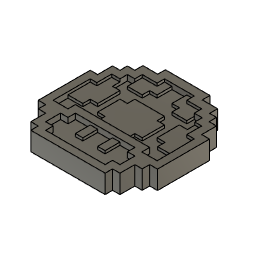
mushroom-8-bit (Autodesk Fusion 360 design; units mm, degrees)
Autodesk Fusion 360 part; units mm, degrees
sketch "Limit" plane through (0, 0, 0) normal (0, 0, 1) x (1, 0, 0)
  line L0 (0, 0) -> (70, 0)
  line L1 (70, 0) -> (70, 100)
  line L2 (70, 100) -> (0, 100)
  line L3 (0, 100) -> (0, 0)
  constraint horizontal L0
  constraint vertical L1
  constraint horizontal L2
  constraint vertical L3
  constraint coincident L0.start L3.end
sketch "Mushroom Head" plane through (0, 0, 0) normal (0, 0, 1) x (1, 0, 0)
  line L0 (11, 35) -> (11, 27)
  line L1 (11, 27) -> (15, 27)
  line L2 (15, 27) -> (15, 23)
  line L3 (15, 23) -> (55, 23)
  line L4 (55, 23) -> (55, 27)
  line L5 (55, 27) -> (59, 27)
  line L6 (59, 27) -> (59, 35)
  line L7 (59, 35) -> (63, 35)
  line L8 (63, 35) -> (63, 39)
  line L9 (63, 39) -> (67, 39)
  line L10 (67, 39) -> (67.2, 39)
  line L11 (67.2, 39) -> (67.2, 67)
  line L12 (67.2, 67) -> (63, 67)
  line L13 (63, 67) -> (63, 75)
  line L14 (63, 75) -> (59, 75)
  line L15 (59, 75) -> (59, 79)
  line L16 (59, 79) -> (55.2513, 79)
  line L17 (55.2513, 79) -> (55.2513, 83.3387)
  line L18 (55.2513, 83.3387) -> (47, 83.3387)
  line L19 (47, 83.3387) -> (47, 87.463)
  line L20 (47, 87.463) -> (23, 87.463)
  line L21 (23, 87.463) -> (23, 83.3387)
  line L22 (23, 83.3387) -> (15, 83.3387)
  line L23 (15, 83.3387) -> (15, 79)
  line L24 (15, 79) -> (11, 79)
  line L25 (11, 79) -> (11, 75)
  line L26 (11, 75) -> (7, 75)
  line L27 (7, 75) -> (7, 67)
  line L28 (7, 67) -> (3, 67)
  line L29 (3, 67) -> (3, 39)
  line L30 (3, 39) -> (7, 39)
  line L31 (7, 39) -> (7, 35)
  line L32 (7, 35) -> (11, 35)
  constraint vertical L0
  constraint perpendicular L0 L1
  constraint perpendicular L1 L2
  constraint perpendicular L0 L3
  constraint perpendicular L3 L4
  constraint perpendicular L0 L5
  constraint perpendicular L5 L6
  constraint perpendicular L6 L7
  constraint perpendicular L7 L8
  constraint perpendicular L8 L9
  constraint perpendicular L8 L10
  constraint perpendicular L9 L11
  constraint perpendicular L8 L12
  constraint perpendicular L9 L13
  constraint perpendicular L13 L14
  constraint perpendicular L14 L15
  constraint perpendicular L15 L16
  constraint perpendicular L16 L17
  constraint perpendicular L17 L18
  constraint perpendicular L18 L19
  constraint perpendicular L19 L20
  constraint perpendicular L20 L21
  constraint perpendicular L21 L22
  constraint perpendicular L16 L23
  constraint perpendicular L23 L24
  constraint perpendicular L14 L25
  constraint perpendicular L25 L26
  constraint perpendicular L14 L27
  constraint perpendicular L27 L28
  constraint perpendicular L14 L29
  constraint perpendicular L29 L30
  constraint perpendicular L30 L31
  constraint perpendicular L0 L32
extrude "Extrude2" add sketch "Mushroom Head" along normal blind 10
sketch "Mushroom Red Front" plane through (0, 0, 10) normal (0, 0, 1) x (-1, 0, 0)
  line L0 (-7, -35) -> (-11, -35)
  line L1 (-11, -35) -> (-11, -27)
  line L2 (-11, -27) -> (-15, -27)
  line L3 (-15, -27) -> (-15, -23)
  line L4 (-15, -23) -> (-55, -23)
  line L5 (-55, -23) -> (-55, -27)
  line L6 (-55, -27) -> (-59, -27)
  line L7 (-59, -27) -> (-59, -35)
  line L8 (-59, -35) -> (-63, -35)
  line L9 (-63, -35) -> (-63, -39)
  line L10 (-63, -39) -> (-67.2, -39)
  line L11 (-67.2, -39) -> (-67.2, -67)
  line L12 (-67.2, -67) -> (-63, -67)
  line L13 (-63, -67) -> (-63, -75)
  line L14 (-63, -75) -> (-59, -75)
  line L15 (-59, -75) -> (-59, -79)
  line L16 (-59, -79) -> (-55.2513, -79)
  line L17 (-55.2513, -79) -> (-55.2513, -83.3387)
  line L18 (-55.2513, -83.3387) -> (-47, -83.3387)
  line L19 (-47, -83.3387) -> (-47, -87.463)
  line L20 (-47, -87.463) -> (-23, -87.463)
  line L21 (-23, -87.463) -> (-23, -83.3387)
  line L22 (-23, -83.3387) -> (-15, -83.3387)
  line L23 (-15, -83.3387) -> (-15, -79)
  line L24 (-15, -79) -> (-11, -79)
  line L25 (-11, -79) -> (-11, -75)
  line L26 (-11, -75) -> (-7, -75)
  line L27 (-7, -75) -> (-7, -67)
  line L28 (-7, -67) -> (-3, -67)
  line L29 (-3, -67) -> (-3, -39)
  line L30 (-3, -39) -> (-7, -39)
  line L31 (-7, -39) -> (-7, -35)
  line L32 (-15, -51) -> (-7, -51)
  line L33 (-7, -51) -> (-7, -43)
  line L34 (-7, -43) -> (-15, -43)
  line L35 (-15, -43) -> (-15, -47)
  line L36 (-15, -47) -> (-27, -47)
  line L37 (-27, -47) -> (-27, -51)
  line L38 (-27, -51) -> (-23, -51)
  line L39 (-23, -51) -> (-23, -63)
  line L40 (-23, -63) -> (-27, -63)
  line L41 (-27, -63) -> (-27, -67)
  line L42 (-27, -67) -> (-43, -67)
  line L43 (-43, -67) -> (-43, -63)
  line L44 (-43, -63) -> (-47, -63)
  line L45 (-47, -63) -> (-47, -51)
  line L46 (-47, -51) -> (-43, -51)
  line L47 (-43, -51) -> (-43, -47)
  line L48 (-43, -47) -> (-55, -47)
  line L49 (-55, -47) -> (-55, -42.8038)
  line L50 (-55, -42.8038) -> (-63.1993, -42.8038)
  line L51 (-63.1993, -42.8038) -> (-63.1993, -51)
  line L52 (-63.1993, -51) -> (-55.2638, -51)
  line L53 (-55.2638, -51) -> (-55.2638, -55)
  line L54 (-55.2638, -55) -> (-51, -55)
  line L55 (-51, -55) -> (-51, -67)
  line L56 (-51, -67) -> (-55.2638, -67)
  line L57 (-55.2638, -67) -> (-55.2638, -75)
  line L58 (-55.2638, -75) -> (-51, -75)
  line L59 (-51, -75) -> (-51, -71)
  line L60 (-51, -71) -> (-43, -71)
  line L61 (-43, -71) -> (-43, -75)
  line L62 (-43, -75) -> (-39, -75)
  line L63 (-39, -75) -> (-39, -83)
  line L64 (-39, -83) -> (-31, -83)
  line L65 (-31, -83) -> (-31, -75)
  line L66 (-31, -75) -> (-27, -75)
  line L67 (-27, -75) -> (-27, -71)
  line L68 (-27, -71) -> (-19, -71)
  line L69 (-19, -71) -> (-19, -75)
  line L70 (-19, -75) -> (-15, -75)
  line L71 (-15, -75) -> (-15, -67)
  line L72 (-15, -67) -> (-19, -67)
  line L73 (-19, -67) -> (-19, -55)
  line L74 (-19, -55) -> (-15, -55)
  line L75 (-15, -55) -> (-15, -51)
  constraint parallel L28 L32
  constraint perpendicular L32 L33
  constraint perpendicular L33 L34
  constraint perpendicular L34 L35
  constraint perpendicular L35 L36
  constraint perpendicular L34 L37
  constraint perpendicular L37 L38
  constraint perpendicular L38 L39
  constraint perpendicular L39 L40
  constraint perpendicular L40 L41
  constraint perpendicular L41 L42
  constraint perpendicular L42 L43
  constraint perpendicular L43 L44
  constraint perpendicular L44 L45
  constraint perpendicular L45 L46
  constraint perpendicular L46 L47
  constraint perpendicular L45 L48
  constraint perpendicular L48 L49
  constraint perpendicular L49 L50
  constraint perpendicular L50 L51
  constraint perpendicular L51 L52
  constraint perpendicular L52 L53
  constraint perpendicular L51 L54
  constraint perpendicular L54 L55
  constraint perpendicular L55 L56
  constraint perpendicular L56 L57
  constraint perpendicular L55 L58
  constraint perpendicular L58 L59
  constraint perpendicular L59 L60
  constraint perpendicular L60 L61
  constraint perpendicular L61 L62
  constraint perpendicular L62 L63
  constraint perpendicular L63 L64
  constraint perpendicular L64 L65
  constraint perpendicular L63 L66
  constraint perpendicular L66 L67
  constraint perpendicular L67 L68
  constraint perpendicular L68 L69
  constraint perpendicular L69 L70
  constraint perpendicular L70 L71
  constraint perpendicular L71 L72
  constraint perpendicular L72 L73
  constraint perpendicular L73 L74
  constraint perpendicular L32 L75
extrude "Extrude3" cut sketch "Mushroom Red Front" against normal blind 3 contours L32 L33 L34 L35 L36 L37 L38 L39 L40 L41 L42 L43 L44 L45 L46 L47 L48 L49 L50 L51 L52 L53 L54 L55 L56 L57 L58 L59 L60 L61 L62 L63 L64 L65 L66 L67 L68 L69 L70 L71 L72 L73 L74 L75
sketch "Mushroom White Front" plane through (0, 0, 10) normal (0, 0, 1) x (-1, 0, 0)
  line L0 (-7, -51) -> (-15, -51)
  line L1 (-15, -51) -> (-15, -55)
  line L2 (-15, -55) -> (-19, -55)
  line L3 (-19, -55) -> (-19, -67)
  line L4 (-19, -67) -> (-15, -67)
  line L5 (-15, -67) -> (-15, -75)
  line L6 (-15, -75) -> (-19, -75)
  line L7 (-19, -75) -> (-19, -71)
  line L8 (-19, -71) -> (-27, -71)
  line L9 (-27, -71) -> (-27, -75)
  line L10 (-27, -75) -> (-31, -75)
  line L11 (-31, -75) -> (-31, -83)
  line L12 (-31, -83) -> (-39, -83)
  line L13 (-39, -83) -> (-39, -75)
  line L14 (-39, -75) -> (-43, -75)
  line L15 (-43, -75) -> (-43, -71)
  line L16 (-43, -71) -> (-51, -71)
  line L17 (-51, -71) -> (-51, -75)
  line L18 (-51, -75) -> (-55.2638, -75)
  line L19 (-55.2638, -75) -> (-55.2638, -67)
  line L20 (-55.2638, -67) -> (-51, -67)
  line L21 (-51, -67) -> (-51, -55)
  line L22 (-51, -55) -> (-55.2638, -55)
  line L23 (-55.2638, -55) -> (-55.2638, -51)
  line L24 (-55.2638, -51) -> (-63.1993, -51)
  line L25 (-63.1993, -51) -> (-63.1993, -42.8038)
  line L26 (-63.1993, -42.8038) -> (-55, -42.8038)
  line L27 (-55, -42.8038) -> (-55, -47)
  line L28 (-55, -47) -> (-43, -47)
  line L29 (-43, -47) -> (-43, -51)
  line L30 (-43, -51) -> (-47, -51)
  line L31 (-47, -51) -> (-47, -63)
  line L32 (-47, -63) -> (-43, -63)
  line L33 (-43, -63) -> (-43, -67)
  line L34 (-43, -67) -> (-27, -67)
  line L35 (-27, -67) -> (-27, -63)
  line L36 (-27, -63) -> (-23, -63)
  line L37 (-23, -63) -> (-23, -51)
  line L38 (-23, -51) -> (-27, -51)
  line L39 (-27, -51) -> (-27, -47)
  line L40 (-27, -47) -> (-15, -47)
  line L41 (-15, -47) -> (-15, -43)
  line L42 (-15, -43) -> (-7, -43)
  line L43 (-7, -43) -> (-7, -51)
  line L44 (-7, -35) -> (-11, -35)
  line L45 (-11, -35) -> (-11, -27)
  line L46 (-11, -27) -> (-15, -27)
  line L47 (-15, -27) -> (-15, -23)
  line L48 (-15, -23) -> (-55, -23)
  line L49 (-55, -23) -> (-55, -27)
  line L50 (-55, -27) -> (-59, -27)
  line L51 (-59, -27) -> (-59, -35)
  line L52 (-59, -35) -> (-63, -35)
  line L53 (-63, -35) -> (-63, -39)
  line L54 (-63, -39) -> (-67.2, -39)
  line L55 (-67.2, -39) -> (-67.2, -67)
  line L56 (-67.2, -67) -> (-63, -67)
  line L57 (-63, -67) -> (-63, -75)
  line L58 (-63, -75) -> (-59, -75)
  line L59 (-59, -75) -> (-59, -79)
  line L60 (-59, -79) -> (-55.2513, -79)
  line L61 (-55.2513, -79) -> (-55.2513, -83.3387)
  line L62 (-55.2513, -83.3387) -> (-47, -83.3387)
  line L63 (-47, -83.3387) -> (-47, -87.463)
  line L64 (-47, -87.463) -> (-23, -87.463)
  line L65 (-23, -87.463) -> (-23, -83.3387)
  line L66 (-23, -83.3387) -> (-15, -83.3387)
  line L67 (-15, -83.3387) -> (-15, -79)
  line L68 (-15, -79) -> (-11, -79)
  line L69 (-11, -79) -> (-11, -75)
  line L70 (-11, -75) -> (-7, -75)
  line L71 (-7, -75) -> (-7, -67)
  line L72 (-7, -67) -> (-3, -67)
  line L73 (-3, -67) -> (-3, -39)
  line L74 (-3, -39) -> (-7, -39)
  line L75 (-7, -39) -> (-7, -35)
  line L76 (-27, -63) -> (-23, -63)
  line L77 (-23, -51) -> (-27, -51)
  line L78 (-27, -47) -> (-43, -47)
  line L79 (-43, -51) -> (-47, -51)
  line L80 (-47, -63) -> (-43, -63)
  line L81 (-43, -67) -> (-27, -67)
  line L82 (-27, -63) -> (-27, -67)
  line L83 (-55.2638, -71) -> (-59, -71)
  line L84 (-59, -71) -> (-59, -63)
  line L85 (-59, -63) -> (-63, -63)
  line L86 (-63, -63) -> (-63.1993, -51)
  line L87 (-55.2638, -51) -> (-55.2638, -55)
  line L88 (-51, -55) -> (-51, -67)
  line L89 (-55.2638, -67) -> (-55.2638, -71)
  line L90 (-15, -71) -> (-10.5513, -71)
  line L91 (-10.5513, -71) -> (-10.5513, -63)
  line L92 (-10.5513, -63) -> (-7, -63)
  line L93 (-7, -63) -> (-7, -51)
  line L94 (-15, -51) -> (-15, -55)
  line L95 (-19, -55) -> (-19, -67)
  line L96 (-15, -67) -> (-15, -71)
  line L97 (-19, -71) -> (-27, -71)
  line L98 (-27, -75) -> (-31, -75)
  line L99 (-31, -83) -> (-27, -83)
  line L100 (-27, -83) -> (-27, -79)
  line L101 (-27, -79) -> (-19, -79)
  line L102 (-19, -79) -> (-19, -71)
  line L103 (-39, -83) -> (-43, -83)
  line L104 (-43, -83) -> (-43, -79)
  line L105 (-43, -79) -> (-51, -79)
  line L106 (-51, -79) -> (-51, -71)
  line L107 (-43, -71) -> (-43, -75)
  line L108 (-39, -75) -> (-39, -83)
  constraint coincident L35.end L36.start
  constraint coincident L36.end L37.start
  constraint coincident L37.end L38.start
  constraint coincident L38.end L39.start
  constraint coincident L39.end L40.start
  constraint coincident L28.end L29.start
  constraint coincident L29.end L30.start
  constraint coincident L30.end L31.start
  constraint coincident L31.end L32.start
  constraint coincident L32.end L33.start
  constraint coincident L33.end L34.start
  constraint coincident L34.end L35.start
  constraint midpoint L19 L83.start
  constraint perpendicular L19 L83
  constraint perpendicular L83 L84
  constraint perpendicular L84 L85
  constraint coincident L24.end L25.start
  constraint coincident L23.end L24.start
  constraint coincident L22.end L23.start
  constraint coincident L21.end L22.start
  constraint coincident L20.end L21.start
  constraint coincident L19.end L20.start
  constraint midpoint L5 L90.start
  constraint perpendicular L5 L90
  constraint perpendicular L90 L91
  constraint perpendicular L91 L92
  constraint coincident L0.start L43.end
  constraint perpendicular L0 L93
  constraint coincident L0.end L1.start
  constraint coincident L1.end L2.start
  constraint coincident L2.end L3.start
  constraint coincident L3.end L4.start
  constraint coincident L4.end L5.start
  constraint coincident L7.end L8.start
  constraint coincident L8.end L9.start
  constraint coincident L9.end L10.start
  constraint coincident L10.end L11.start
  constraint coincident L11.end L12.start
  constraint perpendicular L11 L99
  constraint perpendicular L99 L100
  constraint perpendicular L100 L101
  constraint perpendicular L8 L102
  constraint coincident L12.end L13.start
  constraint perpendicular L13 L103
  constraint perpendicular L103 L104
  constraint perpendicular L104 L105
  constraint coincident L16.end L17.start
  constraint perpendicular L16 L106
  constraint coincident L15.end L16.start
  constraint coincident L14.end L15.start
  constraint coincident L13.end L14.start
sketch "Face Front" plane through (0, 0, 10) normal (0, 0, 1) x (-1, 0, 0)
  line L0 (-55, -31) -> (-55, -39)
  line L1 (-55, -39) -> (-51, -39)
  line L2 (-51, -39) -> (-51, -43)
  line L3 (-51, -43) -> (-43, -43)
  line L4 (-43, -43) -> (-43, -35)
  line L5 (-43, -35) -> (-39, -35)
  line L6 (-39, -35) -> (-39, -43)
  line L7 (-39, -43) -> (-31, -43)
  line L8 (-31, -43) -> (-31, -35)
  line L9 (-31, -35) -> (-27, -35)
  line L10 (-27, -35) -> (-27, -43)
  line L11 (-27, -43) -> (-19, -43)
  line L12 (-19, -43) -> (-19, -39)
  line L13 (-19, -39) -> (-15, -39)
  line L14 (-15, -39) -> (-15, -31)
  line L15 (-15, -31) -> (-19, -31)
  line L16 (-19, -31) -> (-19, -27)
  line L17 (-19, -27) -> (-51, -27)
  line L18 (-51, -27) -> (-51, -31)
  line L19 (-51, -31) -> (-55, -31)
  constraint vertical L0
  constraint perpendicular L0 L1
  constraint perpendicular L1 L2
  constraint perpendicular L0 L3
  constraint perpendicular L3 L4
  constraint perpendicular L4 L5
  constraint perpendicular L5 L6
  constraint perpendicular L6 L7
  constraint perpendicular L7 L8
  constraint perpendicular L8 L9
  constraint perpendicular L9 L10
  constraint perpendicular L10 L11
  constraint perpendicular L11 L12
  constraint perpendicular L10 L13
  constraint perpendicular L13 L14
  constraint perpendicular L14 L15
  constraint perpendicular L15 L16
  constraint perpendicular L16 L17
  constraint perpendicular L17 L18
  constraint perpendicular L0 L19
extrude "Extrude4" cut sketch "Mushroom White Front" against normal blind 1.5 contours L0 L1 L2 L3 L4 L5 L90 L91 L92 L93 L94 L95 L96 | L29 L30 L31 L32 L33 L34 L35 L36 L37 L38 L39 L76 L77 L78 L79 L80 L81 L82 | L7 L8 L9 L10 L11 L97 L98 L99 L100 L101 L102 | L19 L20 L21 L22 L23 L24 L83 L84 L85 L86 L87 L88 L89 | L13 L14 L15 L16 L17 L103 L104 L105 L106 L107 L108
extrude "Extrude5" cut sketch "Face Front" against normal blind 3
sketch "Eyes Front" plane through (0, 0, 10) normal (0, 0, 1) x (-1, 0, 0)
  line L0 (-55, -39) -> (-55, -31)
  line L1 (-55, -31) -> (-51, -31)
  line L2 (-51, -31) -> (-51, -27)
  line L3 (-51, -27) -> (-19, -27)
  line L4 (-19, -27) -> (-19, -31)
  line L5 (-19, -31) -> (-15, -31)
  line L6 (-15, -31) -> (-15, -39)
  line L7 (-15, -39) -> (-19, -39)
  line L8 (-19, -39) -> (-19, -43)
  line L9 (-19, -43) -> (-27, -43)
  line L10 (-27, -43) -> (-27, -35)
  line L11 (-27, -35) -> (-31, -35)
  line L12 (-31, -35) -> (-31, -43)
  line L13 (-31, -43) -> (-39, -43)
  line L14 (-39, -43) -> (-39, -35)
  line L15 (-39, -35) -> (-43, -35)
  line L16 (-43, -35) -> (-43, -43)
  line L17 (-43, -43) -> (-51, -43)
  line L18 (-51, -43) -> (-51, -39)
  line L19 (-51, -39) -> (-55, -39)
  line L20 (-7, -35) -> (-11, -35)
  line L21 (-11, -35) -> (-11, -27)
  line L22 (-11, -27) -> (-15, -27)
  line L23 (-15, -27) -> (-15, -23)
  line L24 (-15, -23) -> (-55, -23)
  line L25 (-55, -23) -> (-55, -27)
  line L26 (-55, -27) -> (-59, -27)
  line L27 (-59, -27) -> (-59, -35)
  line L28 (-59, -35) -> (-63, -35)
  line L29 (-63, -35) -> (-63, -39)
  line L30 (-63, -39) -> (-67.2, -39)
  line L31 (-67.2, -39) -> (-67.2, -67)
  line L32 (-67.2, -67) -> (-63, -67)
  line L33 (-63, -67) -> (-63, -75)
  line L34 (-63, -75) -> (-59, -75)
  line L35 (-59, -75) -> (-59, -79)
  line L36 (-59, -79) -> (-55.2513, -79)
  line L37 (-55.2513, -79) -> (-55.2513, -83.3387)
  line L38 (-55.2513, -83.3387) -> (-47, -83.3387)
  line L39 (-47, -83.3387) -> (-47, -87.463)
  line L40 (-47, -87.463) -> (-23, -87.463)
  line L41 (-23, -87.463) -> (-23, -83.3387)
  line L42 (-23, -83.3387) -> (-15, -83.3387)
  line L43 (-15, -83.3387) -> (-15, -79)
  line L44 (-15, -79) -> (-11, -79)
  line L45 (-11, -79) -> (-11, -75)
  line L46 (-11, -75) -> (-7, -75)
  line L47 (-7, -75) -> (-7, -67)
  line L48 (-7, -67) -> (-3, -67)
  line L49 (-3, -67) -> (-3, -39)
  line L50 (-3, -39) -> (-7, -39)
  line L51 (-7, -39) -> (-7, -35)
  line L52 (-55.2638, -71) -> (-59, -71)
  line L53 (-59, -71) -> (-59, -63)
  line L54 (-59, -63) -> (-63, -63)
  line L55 (-63, -63) -> (-63.1993, -51)
  line L56 (-63.1993, -51) -> (-63.1993, -42.8038)
  line L57 (-63.1993, -42.8038) -> (-55, -42.8038)
  line L58 (-55, -42.8038) -> (-55, -47)
  line L59 (-55, -47) -> (-15, -47)
  line L60 (-15, -47) -> (-15, -43)
  line L61 (-15, -43) -> (-7, -43)
  line L62 (-7, -43) -> (-7, -63)
  line L63 (-7, -63) -> (-10.5513, -63)
  line L64 (-10.5513, -63) -> (-10.5513, -71)
  line L65 (-10.5513, -71) -> (-15, -71)
  line L66 (-15, -71) -> (-15, -75)
  line L67 (-15, -75) -> (-19, -75)
  line L68 (-19, -75) -> (-19, -79)
  line L69 (-19, -79) -> (-27, -79)
  line L70 (-27, -79) -> (-27, -83)
  line L71 (-27, -83) -> (-43, -83)
  line L72 (-43, -83) -> (-43, -79)
  line L73 (-43, -79) -> (-51, -79)
  line L74 (-51, -79) -> (-51, -75)
  line L75 (-51, -75) -> (-55.2638, -75)
  line L76 (-55.2638, -75) -> (-55.2638, -71)
  line L77 (-27, -43) -> (-31, -43)
  line L78 (-31, -43) -> (-31, -35)
  line L79 (-31, -35) -> (-27, -35)
  line L80 (-27, -35) -> (-27, -43)
  line L81 (-39, -43) -> (-43, -43)
  line L82 (-43, -43) -> (-43, -35)
  line L83 (-43, -35) -> (-39, -35)
  line L84 (-39, -35) -> (-39, -43)
  constraint horizontal L77
  constraint vertical L78
  constraint horizontal L79
  constraint vertical L80
  constraint coincident L11.end L12.start
  constraint coincident L9.end L10.start
  constraint horizontal L81
  constraint vertical L82
  constraint horizontal L83
  constraint vertical L84
  constraint coincident L15.end L16.start
  constraint coincident L13.end L14.start
extrude "Extrude6" cut sketch "Eyes Front" against normal blind 1.5 contours L14 L15 L16 L81 L82 L83 L84 | L10 L11 L12 L77 L78 L79 L80
sketch "Mushroom Red Back" plane through (0, 0, 0) normal (0, 0, -1) x (1, 0, 0)
  line L0 (11, -35) -> (7, -35)
  line L1 (7, -35) -> (7, -39)
  line L2 (7, -39) -> (3, -39)
  line L3 (3, -39) -> (3, -67)
  line L4 (3, -67) -> (7, -67)
  line L5 (7, -67) -> (7, -75)
  line L6 (7, -75) -> (11, -75)
  line L7 (11, -75) -> (11, -79)
  line L8 (11, -79) -> (15, -79)
  line L9 (15, -79) -> (15, -83.3387)
  line L10 (15, -83.3387) -> (23, -83.3387)
  line L11 (23, -83.3387) -> (23, -87.463)
  line L12 (23, -87.463) -> (47, -87.463)
  line L13 (47, -87.463) -> (47, -83.3387)
  line L14 (47, -83.3387) -> (55.2513, -83.3387)
  line L15 (55.2513, -83.3387) -> (55.2513, -79)
  line L16 (55.2513, -79) -> (59, -79)
  line L17 (59, -79) -> (59, -75)
  line L18 (59, -75) -> (63, -75)
  line L19 (63, -75) -> (63, -67)
  line L20 (63, -67) -> (67.2, -67)
  line L21 (67.2, -67) -> (67.2, -39)
  line L22 (67.2, -39) -> (63, -39)
  line L23 (63, -39) -> (63, -35)
  line L24 (63, -35) -> (59, -35)
  line L25 (59, -35) -> (59, -27)
  line L26 (59, -27) -> (55, -27)
  line L27 (55, -27) -> (55, -23)
  line L28 (55, -23) -> (15, -23)
  line L29 (15, -23) -> (15, -27)
  line L30 (15, -27) -> (11, -27)
  line L31 (11, -27) -> (11, -35)
  line L32 (55, -71) -> (55, -67)
  line L33 (55, -67) -> (51, -67)
  line L34 (51, -67) -> (51, -55)
  line L35 (51, -55) -> (55, -55)
  line L36 (55, -55) -> (55, -51)
  line L37 (55, -51) -> (63, -51)
  line L38 (63, -51) -> (63, -42.7565)
  line L39 (63, -42.7565) -> (55, -42.7565)
  line L40 (55, -42.7565) -> (55, -46.8783)
  line L41 (55, -46.8783) -> (43, -46.8783)
  line L42 (43, -46.8783) -> (43, -51)
  line L43 (43, -51) -> (47, -51)
  line L44 (47, -51) -> (47, -63)
  line L45 (47, -63) -> (43, -63)
  line L46 (43, -63) -> (43, -67)
  line L47 (43, -67) -> (27, -67)
  line L48 (27, -67) -> (27, -63)
  line L49 (27, -63) -> (23, -63)
  line L50 (23, -63) -> (23, -51)
  line L51 (23, -51) -> (27, -51)
  line L52 (27, -51) -> (27, -47)
  line L53 (27, -47) -> (15, -47)
  line L54 (15, -47) -> (15, -43)
  line L55 (15, -43) -> (7, -43)
  line L56 (7, -43) -> (7, -51)
  line L57 (7, -51) -> (15, -51)
  line L58 (15, -51) -> (15, -55)
  line L59 (15, -55) -> (19, -55)
  line L60 (19, -55) -> (19, -67)
  line L61 (19, -67) -> (15, -67)
  line L62 (15, -67) -> (15, -75)
  line L63 (15, -75) -> (19, -75)
  line L64 (19, -75) -> (19, -71)
  line L65 (19, -71) -> (27, -71)
  line L66 (27, -71) -> (27, -75)
  line L67 (27, -75) -> (31, -75)
  line L68 (31, -75) -> (31, -83)
  line L69 (31, -83) -> (39, -83)
  line L70 (39, -83) -> (39, -75)
  line L71 (39, -75) -> (43, -75)
  line L72 (43, -75) -> (43, -71)
  line L73 (43, -71) -> (51, -71)
  line L74 (51, -71) -> (51, -75)
  line L75 (55, -71) -> (55, -75)
  line L76 (55, -75) -> (51, -75)
  constraint perpendicular L18 L32
  constraint perpendicular L32 L33
  constraint perpendicular L33 L34
  constraint perpendicular L34 L35
  constraint perpendicular L35 L36
  constraint perpendicular L34 L37
  constraint perpendicular L35 L38
  constraint perpendicular L38 L39
  constraint perpendicular L39 L40
  constraint perpendicular L40 L41
  constraint perpendicular L39 L42
  constraint perpendicular L42 L43
  constraint perpendicular L39 L44
  constraint perpendicular L44 L45
  constraint perpendicular L45 L46
  constraint perpendicular L46 L47
  constraint perpendicular L47 L48
  constraint perpendicular L48 L49
  constraint perpendicular L49 L50
  constraint perpendicular L48 L51
  constraint perpendicular L51 L52
  constraint perpendicular L52 L53
  constraint perpendicular L53 L54
  constraint perpendicular L52 L55
  constraint perpendicular L53 L56
  constraint perpendicular L56 L57
  constraint perpendicular L57 L58
  constraint perpendicular L58 L59
  constraint perpendicular L59 L60
  constraint perpendicular L60 L61
  constraint perpendicular L59 L62
  constraint perpendicular L62 L63
  constraint perpendicular L63 L64
  constraint perpendicular L62 L65
  constraint perpendicular L65 L66
  constraint perpendicular L66 L67
  constraint perpendicular L67 L68
  constraint perpendicular L68 L69
  constraint perpendicular L69 L70
  constraint perpendicular L70 L71
  constraint perpendicular L69 L72
  constraint perpendicular L70 L73
  constraint perpendicular L73 L74
  constraint parallel L32 L75
  constraint perpendicular L74 L76
extrude "Extrude7" cut sketch "Mushroom Red Back" against normal blind 3 contours L32 L33 L34 L35 L36 L37 L38 L39 L40 L41 L42 L43 L44 L45 L46 L47 L48 L49 L50 L51 L52 L53 L54 L55 L56 L57 L58 L59 L60 L61 L62 L63 L64 L65 L66 L67 L68 L69 L70 L71 L72 L73 L74 L75 L76
sketch "Mushroom White Back" plane through (0, 0, 0) normal (0, 0, -1) x (1, 0, 0)
  line L0 (51, -67) -> (55, -67)
  line L1 (55, -67) -> (55, -75)
  line L2 (55, -75) -> (51, -75)
  line L3 (51, -75) -> (51, -71)
  line L4 (51, -71) -> (43, -71)
  line L5 (43, -71) -> (43, -75)
  line L6 (43, -75) -> (39, -75)
  line L7 (39, -75) -> (39, -83)
  line L8 (39, -83) -> (31, -83)
  line L9 (31, -83) -> (31, -75)
  line L10 (31, -75) -> (27, -75)
  line L11 (27, -75) -> (27, -71)
  line L12 (27, -71) -> (19, -71)
  line L13 (19, -71) -> (19, -75)
  line L14 (19, -75) -> (15, -75)
  line L15 (15, -75) -> (15, -67)
  line L16 (15, -67) -> (19, -67)
  line L17 (19, -67) -> (19, -55)
  line L18 (19, -55) -> (15, -55)
  line L19 (15, -55) -> (15, -51)
  line L20 (15, -51) -> (7, -51)
  line L21 (7, -51) -> (7, -43)
  line L22 (7, -43) -> (15, -43)
  line L23 (15, -43) -> (15, -47)
  line L24 (15, -47) -> (27, -47)
  line L25 (27, -47) -> (27, -51)
  line L26 (27, -51) -> (23, -51)
  line L27 (23, -51) -> (23, -63)
  line L28 (23, -63) -> (27, -63)
  line L29 (27, -63) -> (27, -67)
  line L30 (27, -67) -> (43, -67)
  line L31 (43, -67) -> (43, -63)
  line L32 (43, -63) -> (47, -63)
  line L33 (47, -63) -> (47, -51)
  line L34 (47, -51) -> (43, -51)
  line L35 (43, -51) -> (43, -46.8783)
  line L36 (43, -46.8783) -> (55, -46.8783)
  line L37 (55, -46.8783) -> (55, -42.7565)
  line L38 (55, -42.7565) -> (63, -42.7565)
  line L39 (63, -42.7565) -> (63, -51)
  line L40 (63, -51) -> (55, -51)
  line L41 (55, -51) -> (55, -55)
  line L42 (55, -55) -> (51, -55)
  line L43 (51, -55) -> (51, -67)
  line L44 (11, -35) -> (7, -35)
  line L45 (7, -35) -> (7, -39)
  line L46 (7, -39) -> (3, -39)
  line L47 (3, -39) -> (3, -67)
  line L48 (3, -67) -> (7, -67)
  line L49 (7, -67) -> (7, -75)
  line L50 (7, -75) -> (11, -75)
  line L51 (11, -75) -> (11, -79)
  line L52 (11, -79) -> (15, -79)
  line L53 (15, -79) -> (15, -83.3387)
  line L54 (15, -83.3387) -> (23, -83.3387)
  line L55 (23, -83.3387) -> (23, -87.463)
  line L56 (23, -87.463) -> (47, -87.463)
  line L57 (47, -87.463) -> (47, -83.3387)
  line L58 (47, -83.3387) -> (55.2513, -83.3387)
  line L59 (55.2513, -83.3387) -> (55.2513, -79)
  line L60 (55.2513, -79) -> (59, -79)
  line L61 (59, -79) -> (59, -75)
  line L62 (59, -75) -> (63, -75)
  line L63 (63, -75) -> (63, -67)
  line L64 (63, -67) -> (67.2, -67)
  line L65 (67.2, -67) -> (67.2, -39)
  line L66 (67.2, -39) -> (63, -39)
  line L67 (63, -39) -> (63, -35)
  line L68 (63, -35) -> (59, -35)
  line L69 (59, -35) -> (59, -27)
  line L70 (59, -27) -> (55, -27)
  line L71 (55, -27) -> (55, -23)
  line L72 (55, -23) -> (15, -23)
  line L73 (15, -23) -> (15, -27)
  line L74 (15, -27) -> (11, -27)
  line L75 (11, -27) -> (11, -35)
  line L76 (27, -47) -> (27, -51)
  line L77 (23, -51) -> (23, -63)
  line L78 (27, -63) -> (27, -67)
  line L79 (23, -63) -> (27, -63)
  line L80 (27, -67) -> (43, -67)
  line L81 (43, -67) -> (43, -63)
  line L82 (47, -63) -> (43, -63)
  line L83 (43, -51) -> (47, -51)
  line L84 (47, -51) -> (47, -63)
  line L85 (43, -51) -> (43, -46.8783)
  line L86 (27, -47) -> (43, -46.8783)
  line L87 (51, -55) -> (51, -67)
  line L88 (55, -67) -> (51, -67)
  line L89 (55, -67) -> (55, -71)
  line L90 (55, -71) -> (59, -71)
  line L91 (59, -71) -> (59, -63)
  line L92 (59, -63) -> (63, -63)
  line L93 (63, -51) -> (63, -63)
  line L94 (55, -55) -> (55, -51)
  line L95 (63, -51) -> (55, -51)
  line L96 (51, -55) -> (55, -55)
  line L97 (19, -71) -> (19, -79)
  line L98 (27, -79) -> (19, -79)
  line L99 (27, -79) -> (27, -83)
  line L100 (27, -83) -> (31, -83)
  line L101 (31, -83) -> (31, -75)
  line L102 (27, -75) -> (31, -75)
  line L103 (27, -71) -> (27, -75)
  line L104 (19, -71) -> (27, -71)
  line L105 (15, -55) -> (19, -55)
  line L106 (19, -55) -> (19, -67)
  line L107 (19, -67) -> (15, -67)
  line L108 (15, -71) -> (15, -67)
  line L109 (15, -71) -> (11, -71)
  line L110 (11, -71) -> (11, -63)
  line L111 (11, -63) -> (7, -63)
  line L112 (7, -63) -> (7, -51)
  line L113 (7, -51) -> (15, -51)
  line L114 (15, -51) -> (15, -55)
  line L115 (39, -83) -> (43, -83)
  line L116 (43, -79) -> (43, -83)
  line L117 (43, -79) -> (51, -79)
  line L118 (51, -79) -> (51, -71)
  line L119 (51, -71) -> (43, -71)
  line L120 (43, -71) -> (43, -75)
  line L121 (43, -75) -> (39, -75)
  line L122 (39, -75) -> (39, -83)
  constraint coincident L24.end L25.start
  constraint coincident L25.end L26.start
  constraint coincident L26.end L27.start
  constraint coincident L27.end L28.start
  constraint coincident L28.end L29.start
  constraint coincident L29.end L30.start
  constraint coincident L30.end L31.start
  constraint coincident L31.end L32.start
  constraint coincident L32.end L33.start
  constraint coincident L34.end L35.start
  constraint coincident L33.end L34.start
  constraint coincident L35.end L36.start
  constraint coincident L42.end L43.start
  constraint coincident L0.start L43.end
  constraint coincident L0.end L1.start
  constraint midpoint L1 L89.end
  constraint perpendicular L1 L90
  constraint perpendicular L90 L91
  constraint perpendicular L91 L92
  constraint coincident L39.end L40.start
  constraint perpendicular L40 L93
  constraint coincident L41.end L42.start
  constraint coincident L40.end L41.start
  constraint coincident L12.end L13.start
  constraint perpendicular L14 L97
  constraint perpendicular L97 L98
  constraint perpendicular L98 L99
  constraint coincident L8.end L9.start
  constraint perpendicular L99 L100
  constraint coincident L9.end L10.start
  constraint coincident L10.end L11.start
  constraint coincident L11.end L12.start
  constraint coincident L18.end L19.start
  constraint coincident L17.end L18.start
  constraint coincident L16.end L17.start
  constraint coincident L15.end L16.start
  constraint midpoint L15 L108.start
  constraint perpendicular L108 L109
  constraint perpendicular L109 L110
  constraint perpendicular L110 L111
  constraint coincident L20.end L21.start
  constraint perpendicular L20 L112
  constraint coincident L19.end L20.start
  constraint coincident L7.end L8.start
  constraint perpendicular L7 L115
  constraint perpendicular L115 L116
  constraint perpendicular L116 L117
  constraint coincident L3.end L4.start
  constraint perpendicular L4 L118
  constraint coincident L4.end L5.start
  constraint coincident L5.end L6.start
  constraint coincident L6.end L7.start
extrude "Extrude8" cut sketch "Mushroom White Back" against normal blind 1.5 contours L0 L1 L40 L41 L42 L43 L87 L88 L89 L90 L91 L92 L93 L94 L95 L96 | L3 L4 L5 L6 L7 L115 L116 L117 L118 L119 L120 L121 L122 | L25 L26 L27 L28 L29 L30 L31 L32 L33 L34 L35 L76 L77 L78 L79 L80 L81 L82 L83 L84 L85 L86 | L9 L10 L11 L12 L13 L97 L98 L99 L100 L101 L102 L103 L104 | L15 L16 L17 L18 L19 L20 L105 L106 L107 L108 L109 L110 L111 L112 L113 L114
named bodies: "Mushroom"
